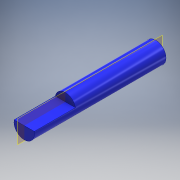
# Autodesk Inventor part: 8mm Shaft
Saved by Autodesk Inventor 2017 (Build 210142000, 142)
## iProperties
Created: 2017-04-29
Part Number: 8mm Shaft
Material: Generic
Document SubType Name: Modeling
Designer: Parshant Bombhi
Density: 1 g/cm^3
Appearance: Blue - Wall Paint - Glossy
Author: Parshant Bombhi
Autodesk Inventor part; units mm, degrees
ref_plane "XZ Plane" through (0, 0, 0) normal (0, 1, 0) x (-1, 0, 0)
ref_plane "XY Plane" through (0, 0, 0) normal (0, 0, 1) x (1, 0, 0)
sketch "Sketch1" plane through (0, 0, 0) normal (0, 1, 0) x (-1, 0, 0)
  circle A0 centre (0, 0) radius 3.9688
  dimension "d0" = 7.9375
  constraints: 1 centre point, 1 coincident
  measures "d0" diameter of A0
extrude "Extrusion1" add sketch "Sketch1" along normal blind 50.8
sketch "Sketch2" plane through (0, 0, 0) normal (1, 0, 0) x (0, 1, 0)
  line L0 (0, 3.9688) -> (0, -3.9688) projected
  line L1 (0, 3.9688) -> (50.8, 3.9688) projected
  line L2 (0, 0.7937) -> (15.875, 0.7937)
  line L3 (15.875, 0.7937) -> (15.875, 3.9688)
  line L4 (15.875, 3.9688) -> (0, 3.9688)
  line L5 (0, 3.9688) -> (0, 0.7937)
  point P0 (0, 0)
  dimension "d3" = 15.875
  dimension "d4" = 3.175
  constraints: 8 end point, 2 parallel, 2 point on line, 1 horizontal, 1 perpendicular
  measures "d3" distance of L2.start L2.end
  measures "d4" distance of L2.end L3.end
extrude "Extrusion2" cut sketch "Sketch2" along normal mid plane 25.4
body "Solid1"
